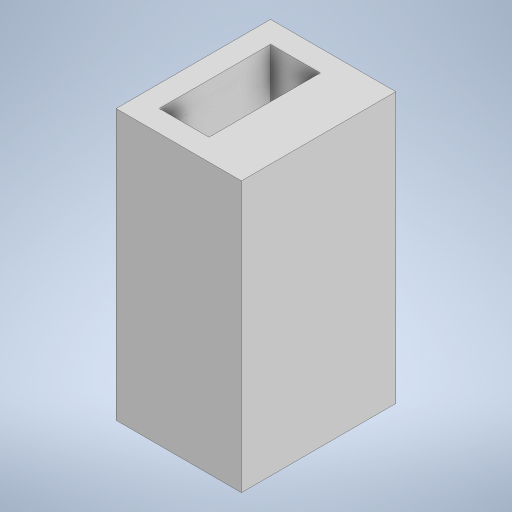
# Autodesk Inventor part: front-camera-support
Saved by Autodesk Inventor 2023 (Build 270158000, 158)
## iProperties
Created: 2024-04-10
Part Number: front-camera-support
Material: Genérico
Document SubType Name: Modeling
Designer: inigo
Density: 1 g/cm^3
Appearance: Valor por defecto
Author: inigo
Autodesk Inventor part; units mm, degrees
ref_plane "YZ Plane" through (0, 0, 0) normal (1, 0, 0) x (0, 1, 0)
ref_plane "XZ Plane" through (0, 0, 0) normal (0, 1, 0) x (-1, 0, 0)
ref_plane "XY Plane" through (0, 0, 0) normal (0, 0, 1) x (1, 0, 0)
sketch "Boceto1" plane through (0, 0, 0) normal (0, 1, 0) x (-1, 0, 0)
  line L0 (2.3, 5.15) -> (-2.3, 5.15)
  line L1 (-2.3, 5.15) -> (-2.3, -5.15)
  line L2 (-2.3, -5.15) -> (2.3, -5.15)
  line L3 (2.3, -5.15) -> (2.3, 5.15)
  line L4 (2.3, 5.15) -> (-2.3, -5.15) construction
  line L5 (-2.3, 5.15) -> (2.3, -5.15) construction
  line L6 (4.3, 7.15) -> (-4.3, 7.15)
  line L7 (-4.3, 7.15) -> (-4.3, -7.15)
  line L8 (-4.3, -7.15) -> (4.3, -7.15)
  line L9 (4.3, -7.15) -> (4.3, 7.15)
  point P0 (0, 0)
  dimension "d0" = 10.3
  dimension "d1" = 4.6
  dimension "d2" = 2
  constraints: 20 end point, 4 parallel, 2 midpoint, 2 perpendicular, 1 horizontal, 3 other
  measures "d0" distance of L1.end L0.end
  measures "d1" distance between parallel lines of L1 L3
  measures "d2" distance between parallel lines of L3 L9
extrude "Extrusión1" add sketch "Boceto1" along normal blind 2 contours L3 L2 L1 L0
sketch "Boceto3" plane through (0, 0, 0) normal (0, -1, 0) x (1, 0, 0)
  line L0 (2.3, -5.15) -> (-2.3, -5.15) projected
  line L1 (-2.3, 5.15) -> (2.3, 5.15)
  line L2 (2.3, 5.15) -> (2.3, -5.15)
  line L3 (2.3, -5.15) -> (-2.3, -5.15)
  line L4 (-2.3, -5.15) -> (-2.3, 5.15)
  line L5 (-2.3, 5.15) -> (2.3, -5.15) construction
  line L6 (2.3, 5.15) -> (-2.3, -5.15) construction
  line L7 (4.3, -7.15) -> (4.3, 7.15)
  line L8 (4.3, 7.15) -> (-4.3, 7.15)
  line L9 (-4.3, 7.15) -> (-4.3, -7.15)
  line L10 (-4.3, -7.15) -> (4.3, -7.15)
  line L11 (2.3, 7.15) -> (7.3, 7.15)
  line L12 (7.3, 7.15) -> (7.3, -7.15)
  line L13 (7.3, -7.15) -> (2.3, -7.15)
  line L14 (2.3, -7.15) -> (2.3, 7.15)
  point P0 (0, 0)
  dimension "d5" = 2
  dimension "d6" = 5
  constraints: 28 end point, 6 parallel, 3 perpendicular, 2 horizontal, 2 midpoint, 1 point on line, 3 other
  measures "d5" distance between parallel lines of L2 L7
  measures "d6" distance of L12.end L13.end
extrude "Extrusión2" add sketch "Boceto3" against normal blind 25 contours L14 L10 L9 L8 L1 L4 L0 | L2 L14 L8 L7 L10 | L7 L11 L12 L13
